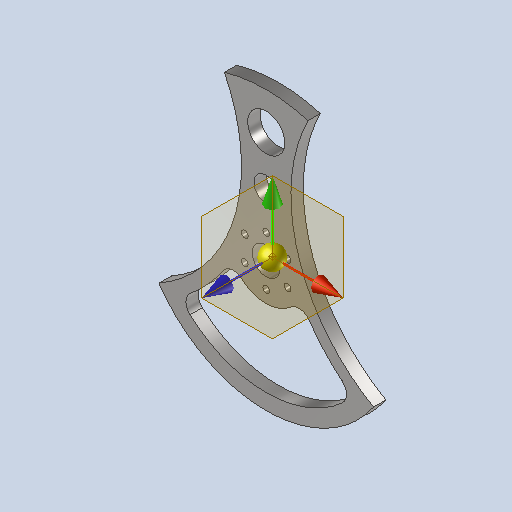
# Autodesk Inventor part: Blade (Bar)
Saved by Autodesk Inventor 2022.3 (Build 263350000, 350)
## iProperties
Created: 2022-06-12
Part Number: Blade (Bar)
Material: Stainless Steel
Document SubType Name: Modeling
Designer: Nathan Cai
Density: 8 g/cm^3
Appearance: Semi-Polished
Mass: 196.473 g
Surface Area: 131.075 cm^2
Volume: 24.5592 cm^3
Author: Nathan Cai
Autodesk Inventor part; units mm, degrees
ref_plane "YZ Plane" through (0, 0, 0) normal (1, 0, 0) x (0, 1, 0)
ref_plane "XZ Plane" through (0, 0, 0) normal (0, 1, 0) x (-1, 0, 0)
ref_plane "XY Plane" through (0, 0, 0) normal (0, 0, 1) x (1, 0, 0)
sketch "Sketch1" plane through (0, 0, 0) normal (0, 0, 1) x (1, 0, 0)
  circle A0 centre (0, 0) radius 7.1437
  line L0 (0, 0) -> (0, 12.7) construction
  circle A1 centre (0, 12.7) radius 1.7526
  circle A2 centre (-10.9985, 6.35) radius 1.7526
  circle A3 centre (-10.9985, -6.35) radius 1.7526
  circle A4 centre (0, -12.7) radius 1.7526
  circle A5 centre (10.9985, -6.35) radius 1.7526
  circle A6 centre (10.9985, 6.35) radius 1.7526
  circle A7 centre (0, 0) radius 76.2 construction
  line L1 (-12.7, -75.1342) -> (12.7, -75.1342) construction
  line L2 (12.7, -75.1342) -> (12.7, 75.1342) construction
  line L3 (12.7, 75.1342) -> (-12.7, 75.1342) construction
  line L4 (-12.7, 75.1342) -> (-12.7, -75.1342) construction
  line L5 (-12.7, -75.1342) -> (12.7, 75.1342) construction
  line L6 (12.7, -75.1342) -> (-12.7, 75.1342) construction
  line L7 (0, 76.2) -> (0, -76.2) construction
  line L8 (0, 0) -> (21.47, 73.1128) construction
  circle A8 centre (0, 0) radius 66.675 construction
  circle A9 centre (0, 0) radius 19.05
  arc A10 (21.47, 73.1128) -> (55.1282, -37.5025) centre (97.0123, 35.6704) ccw
  line L9 (21.47, 73.1128) -> (17.1652, 64.4276) construction
  arc A11 (-55.1282, -37.5025) -> (-21.47, 73.1128) centre (-97.0123, 35.6704) ccw
  arc A12 (21.47, 73.1128) -> (-21.47, 73.1128) centre (0, 0) ccw
  line L10 (-12.7, 0) -> (12.7, 0) construction
  circle A13 centre (0, 57.15) radius 9.525
  circle A14 centre (0, 31.75) radius 6.35
  arc A15 (-55.1282, -37.5025) -> (55.1282, -37.5025) centre (0, 0) ccw
  arc A16 (-44.451, -38.2008) -> (44.451, -38.2008) centre (0, 0) ccw
  arc A17 (-44.451, -38.2008) -> (-17.412, -7.7282) centre (-97.0123, 35.6704) ccw
  arc A18 (17.412, -7.7282) -> (44.451, -38.2008) centre (97.0123, 35.6704) ccw
  point P0 (0, 75.1342)
  point P1 (17.8797, 6.5742)
  point P2 (-17.8797, 6.5742)
  point P3 (0, -66.675)
  dimension "d0" = 14.2875
  dimension "d1" = 12.7
  dimension "d2" = 3.5052
  dimension "d5" = 360
  dimension "d7" = 152.4
  dimension "d8" = 25.4
  dimension "d9" = 9.525
  dimension "d10" = 38.1
  dimension "d11" = 10
  dimension "d12" = 19.05
  dimension "d13" = 57.15
  dimension "d14" = 12.7
  dimension "d15" = 31.75
  dimension "d20" = 6.35
  dimension "d21" = 6.35
  dimension "d22" = 8.0645
  constraints: 30 point on circle, 22 end point, 19 centre point, 7 midpoint, 4 coincident, 3 point on line, 3 symmetric about line, 3 tangent, 2 parallel, 2 perpendicular, 1 concentric, 1 horizontal, 1 vertical, 14 other
  measures "d0" diameter of A0
  measures "d1" distance of L0.start L0.end
  measures "d2" diameter of A1
  measures "d7" diameter of A7
  measures "d8" distance of L3.end L2.end
  measures "d9" radial gap between concentric circles of A7 A8
  measures "d10" diameter of A9
  measures "d11" angle of L9 L8
  measures "d12" diameter of A13
  measures "d13" distance of point (0, 0) A13.centre
  measures "d14" diameter of A14
  measures "d15" distance of point (0, 0) A14.centre
  measures "d20" radial gap between concentric circles of A11 A17
  measures "d21" radial gap between concentric circles of A10 A18
  measures "d22" radial gap between concentric circles of A15 A16
extrude "Extrusion1" add sketch "Sketch1" along normal blind 6.35 contours A9 | A17 A16 A18 A9 A10 A15 A11 | A11 A12 A10 A9
sketch "Sketch2" plane through (0, 0, 6.35) normal (0, 0, 1) x (1, 0, 0)
  arc A0 (21.47, 73.1128) -> (-21.47, 73.1128) centre (0, 0) ccw projected
  line L0 (21.47, 73.1128) -> (-12.8922, 83.2035)
  point P0 (0, 0)
  constraints: 2 end point, 1 tangent
fillet "Fillet1" radius 6.35 4 edges at (-17.412, -7.7282, 3.175) (17.412, -7.7282, 3.175) (44.451, -38.2008, 3.175) (-44.451, -38.2008, 3.175)
equation "\"d21\" = d20"
body "Solid1"
